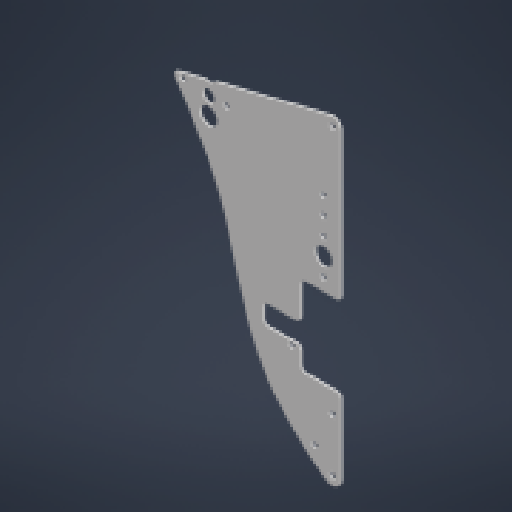
# Autodesk Inventor part: outer-tower-support-proto
Saved by Autodesk Inventor 2023.2 (Build 272271000, 271)
## iProperties
Created: 2023-03-21
Part Number: outer-tower-support-proto
Material: Generic
Document SubType Name: Modeling
Designer: Liam
Density: 1 g/cm^3
Appearance: Default
Author: Liam
Autodesk Inventor part; units mm, degrees
ref_plane "YZ Plane" through (0, 0, 0) normal (1, 0, 0) x (0, 1, 0)
ref_plane "XZ Plane" through (0, 0, 0) normal (0, 1, 0) x (-1, 0, 0)
ref_plane "XY Plane" through (0, 0, 0) normal (0, 0, 1) x (1, 0, 0)
sketch "Sketch1" plane through (0, 0, 0) normal (0, 0, 1) x (1, 0, 0)
  circle A0 centre (-71.4375, -30.1625) radius 6.35
  line L0 (23.8157, 7.5349) -> (23.8157, -44.8526)
  arc A1 (13.7984, -214.7362) -> (23.8125, -209.55) centre (17.4625, -209.55) ccw
  arc A2 (23.8157, 7.5349) -> (15.9224, 14.0979) centre (17.4787, 7.9416) ccw
  circle A3 centre (-71.4375, -17.4625) radius 2.1844
  line L1 (-85.6776, -11.3021) -> (-75.211, -8.6854)
  line L2 (15.9224, 14.0979) -> (-66.2619, -6.4482)
  arc A4 (-73.1895, -8.8477) -> (-67.9692, -7.5426) centre (-71.4375, -4.7625) ccw
  arc A5 (-66.2619, -6.4482) -> (-67.9692, -7.5426) centre (-65.4918, -9.5284) ccw
  arc A6 (-73.1895, -8.8477) -> (-75.211, -8.6854) centre (-74.4409, -11.7656) ccw
  circle A7 centre (-71.4375, -17.4625) radius 4.445
  circle A8 centre (11.1125, -88.9) radius 2.0955
  line L3 (23.8125, -159.2779) -> (23.8125, -209.55)
  line L4 (23.8157, -44.8526) -> (23.8157, -94.965)
  circle A9 centre (17.4787, 7.9416) radius 2.0955
  circle A10 centre (-90.0286, -15.9272) radius 2.1082
  circle A11 centre (-58.7375, -17.4625) radius 2.0955
  circle A12 centre (11.1125, -38.1) radius 2.0955
  circle A13 centre (17.4625, -209.55) radius 2.1082
  circle A14 centre (4.7625, -196.85) radius 2.1082
  line L5 (-1.7875, -155.86) -> (20.6375, -155.86)
  line L6 (23.8125, -159.035) -> (23.8125, -159.2779)
  line L7 (-1.7875, -98.14) -> (20.6407, -98.14)
  arc A15 (-5.5975, -152.05) -> (-1.7875, -155.86) centre (-1.7875, -152.05) ccw
  arc A16 (-1.7875, -98.14) -> (-5.5975, -101.95) centre (-1.7875, -101.95) ccw
  arc A17 (23.8125, -159.035) -> (20.6375, -155.86) centre (20.6375, -159.035) ccw
  arc A18 (20.6407, -98.14) -> (23.8157, -94.965) centre (20.6407, -94.965) ccw
  circle A19 centre (17.4625, -171.45) radius 2.1844
  circle A20 centre (11.1125, -63.5) radius 2.0955
  circle A21 centre (11.1125, -50.8) radius 2.0955
  circle A22 centre (11.1125, -76.2) radius 6.35
  circle A23 centre (-11.5777, -142.9997) radius 2.0955
  line L8 (-29.2746, -140.1414) -> (-8.7725, -140.1414)
  line L9 (-8.7725, -125.8713) -> (-29.2746, -125.8713)
  line L10 (-32.4496, -129.0463) -> (-32.4496, -136.9664)
  line L11 (-5.5975, -143.3164) -> (-5.5975, -152.05)
  line L12 (-5.5975, -122.6963) -> (-5.5975, -101.95)
  arc A24 (-5.5975, -143.3164) -> (-8.7725, -140.1414) centre (-8.7725, -143.3164) ccw
  arc A25 (-8.7725, -125.8713) -> (-5.5975, -122.6963) centre (-8.7725, -122.6963) ccw
  arc A26 (-32.4496, -136.9664) -> (-29.2746, -140.1414) centre (-29.2746, -136.9664) ccw
  arc A27 (-29.2746, -125.8713) -> (-32.4496, -129.0463) centre (-29.2746, -129.0463) ccw
  line L13 (13.7984, -214.7362) -> (12.5183, -213.8318) construction
  line L14 (12.5183, -213.8318) -> (0, -206.2508) construction
  line L15 (0, -206.2508) -> (-17.0986, -187.3696) construction
  line L16 (-17.0986, -187.3696) -> (-31.7765, -172.0523) construction
  line L17 (-31.7765, -172.0523) -> (-45.7993, -138.4697) construction
  line L18 (-45.7993, -138.4697) -> (-54.717, -102.5523) construction
  line L19 (-54.717, -102.5523) -> (-65.0675, -66.1978) construction
  line L20 (-65.0675, -66.1978) -> (-78.5193, -45.4549) construction
  line L21 (-78.5193, -45.4549) -> (-96.3149, -13.9614) construction
  line L22 (-96.3149, -13.9614) -> (-99.8364, -14.8418) construction
  line L23 (-99.8364, -14.8418) -> (-85.6776, -11.3021) construction
  spline S0 degree 4 poles (13.7984, -214.7362) (12.5183, -213.8318) (0, -206.2508) (-17.0986, -187.3696) (-31.7765, -172.0523) (-45.7993, -138.4697) (-54.717, -102.5523) (-65.0675, -66.1978) (-78.5193, -45.4549) (-96.3149, -13.9614) (-99.8364, -14.8418) (-85.6776, -11.3021) knots 1 1 1 1 1 2 3 4 5 6 7 8 9 9 9 9 9
  point P0 (0, 0)
  point P1 (13.9752, -214.8567)
  point P2 (-74.0123, -8.3858)
  point P3 (-67.4605, -6.7478)
  point P4 (23.8125, -209.55)
  dimension "d13" = 12.7
  dimension "d30" = 4.3688
  dimension "d32" = 3.175
  dimension "d33" = 8.89
  dimension "d34" = 4.191
  dimension "d51" = 4.191
  dimension "d52" = 4.2164
  dimension "d54" = 4.2164
  dimension "d55" = 4.2164
  dimension "d62" = 3.175
  dimension "d65" = 4.191
  dimension "d66" = 12.7
  dimension "d67" = 4.191
  dimension "d68" = 4.191
  dimension "d69" = 4.191
  dimension "d71" = 4.191
  dimension "d73" = 3.175
  dimension "d74" = 3.175
  constraints: 29 point on circle, 28 centre point, 26 end point, 16 tangent, 4 equal radius, 4 horizontal, 4 vertical, 3 point on line, 2 coincident, 1 parallel, 1 perpendicular, 23 other
  measures "d13" diameter of A0
  measures "d30" diameter of A3
  measures "d32" radius of A5
  measures "d33" diameter of A7
  measures "d34" diameter of A8
  measures "d51" diameter of A9
  measures "d52" diameter of A10
  measures "d54" diameter of A13
  measures "d55" diameter of A14
  measures "d62" radius of A17
  measures "d65" diameter of A20
  measures "d66" diameter of A22
  measures "d67" diameter of A21
  measures "d68" diameter of A12
  measures "d69" diameter of A11
  measures "d71" diameter of A23
  measures "d73" radius of A24
  measures "d74" radius of A26
extrude "Extrusion7" add sketch "Sketch1" along normal blind 1.524 contours L0 L4 A18 L7 A16 L12 A25 L9 A27 L10 A26 L8 A24 L11 A15 L5 A17 L6 L3 A1 S0 L1 A6 A4 A5 L2 A2
body "Solid7"
